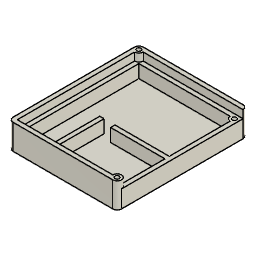
基板外形 (Autodesk Fusion 360 archive; units mm, degrees)
design "筐体A"
Autodesk Fusion 360 part; units mm, degrees
sketch "スケッチ1" plane through (0, 0, 0) normal (0, 0, 1) x (1, 0, 0)
  line L0 (-25, 30) -> (25, 30)
  line L1 (25, 30) -> (25, -30)
  line L2 (25, -30) -> (-25, -30)
  line L3 (-25, -30) -> (-25, 30)
  line L4 (-13.65, 27) -> (13.65, 27)
  line L5 (13.65, 27) -> (13.65, -1.3)
  line L6 (13.65, -1.3) -> (-13.65, -1.3)
  line L7 (-13.65, -1.3) -> (-13.65, 27)
  line L8 (0, 27) -> (0, -1.3)
  line L9 (-7, -6) -> (23, -6)
  line L10 (23, -6) -> (23, -26)
  line L11 (23, -26) -> (-7, -26)
  line L12 (-7, -26) -> (-7, -6)
  line L13 (0, 30) -> (0, -30)
  line L14 (-23, 28) -> (23, 28)
  line L15 (23, 28) -> (23, -28)
  line L16 (23, -28) -> (-23, -28)
  line L17 (-23, -28) -> (-23, 28)
  line L18 (23, 28) -> (25, 28)
  line L19 (23, -28) -> (25, -28)
  circle A0 centre (23, 26) radius 2
  circle A1 centre (23, 26) radius 1
  circle A2 centre (-23, 28) radius 2
  circle A3 centre (-23, 28) radius 1
  circle A4 centre (23, -28) radius 1
  circle A5 centre (23, -28) radius 2
  line L20 (23, -4) -> (-9, -4)
  line L21 (-9, -4) -> (-9, -28)
  line L22 (-9, -28) -> (23, -28)
  line L23 (23, -28) -> (23, -4)
  line L24 (-7, -6) -> (-7, -4)
  line L25 (-2, -6) -> (-2, -4)
  line L26 (-21, 26) -> (23, 26)
  line L27 (23, 26) -> (23, -26)
  line L28 (23, -26) -> (-21, -26)
  line L29 (-21, -26) -> (-21, 26)
  dimension "d1" = 27.3
  dimension "d2" = 28.3
  dimension "d3" = 30
  dimension "d4" = 20
  dimension "d5" = 50
  dimension "d6" = 60
  dimension "d7" = 3
  dimension "d8" = 2
  dimension "d9" = 2
  dimension "d10" = 2
  dimension "d11" = 2
  dimension "d12" = 4
  dimension "d13" = 2
  dimension "d14" = 4
  dimension "d15" = 2
  dimension "d16" = 2
  dimension "d17" = 4
  dimension "d23" = 2
  dimension "d24" = 2
  dimension "d25" = 2
  dimension "d26" = 5
  dimension "d27" = 2
  dimension "d28" = 2
  dimension "d29" = 2
  constraint horizontal L0
  constraint vertical L1
  constraint horizontal L2
  constraint vertical L3
  constraint horizontal L4
  constraint vertical L5
  constraint horizontal L6
  constraint vertical L7
  constraint midpoint L4 L8.start
  constraint midpoint L6 L8.end
  constraint coincident origin L8
  constraint horizontal L9
  constraint vertical L10
  constraint horizontal L11
  constraint vertical L12
  constraint midpoint L0 L13.start
  constraint midpoint L2 L13.end
  constraint midpoint origin L13
  constraint horizontal L14
  constraint vertical L15
  constraint horizontal L16
  constraint vertical L17
  constraint coincident L1 L18.end
  constraint perpendicular L1 L18
  constraint coincident L1 L19.end
  constraint perpendicular L1 L19
  constraint tangent L14 A0
  constraint tangent L1 A0
  constraint concentric A0 A1
  constraint concentric A2 A3
  constraint tangent L0 A2
  constraint tangent L3 A2
  constraint concentric A4 A5
  constraint tangent L1 A5
  constraint tangent L2 A5
  constraint coincident L9.end L15
  constraint horizontal L20
  constraint vertical L21
  constraint horizontal L22
  constraint vertical L23
  constraint coincident L16 L21.end
  constraint coincident L15 L20.start
  constraint coincident L20 L24.end
  constraint perpendicular L20 L24
  constraint coincident L9 L25.start
  constraint coincident L20 L25.end
  constraint perpendicular L20 L25
  constraint horizontal L26
  constraint vertical L27
  constraint horizontal L28
  constraint vertical L29
  constraint collinear L15 L27
  measures "d1" distance of L4.start L4.end
  measures "d2" distance of L4.start L6.end
  measures "d3" distance of L9.start L9.end
  measures "d4" distance of L9.start L11.end
  measures "d5" distance of L0.start L0.end
  measures "d6" distance of L0.end L1.end
  measures "d7" distance of L0 L4
  measures "d8" distance of L3 L17
  measures "d9" distance of L0 L14
  measures "d10" distance of L1 L15
  measures "d11" distance of L2 L16
  measures "d12" diameter of A0
  measures "d13" diameter of A1
  measures "d14" diameter of A2
  measures "d15" diameter of A3
  measures "d16" diameter of A4
  measures "d17" diameter of A5
  measures "d23" distance of L11 L16
  measures "d24" distance of L9 L20
  measures "d25" distance of L12 L21
  measures "d26" distance of L24 L25
  measures "d27" distance of L14 L26
  measures "d28" distance of L17 L29
  measures "d29" distance of L16 L28
extrude "押し出し1" add sketch "スケッチ1" along normal blind 2 contours L0 L13 L14 A2 | L0 L1 L13 L14 L18 | L0 L3 A2 | L14 L17 A2 A3 | L4 L5 L13 L14 A0 L26 | L4 L7 L13 L14 L16 L17 A2 L21 L26 L28 L29 | L1 L18 A0 | L14 L17 A2 A3 | L2 L3 L13 L16 L17 A2 L22 | L4 L7 L8 L13 L26 | L4 L5 L8 L13 L26 | L15 A0 A1 L27 | L15 A0 A1 L26 | L1 L10 L15 A0 A5 L23 L27 | L5 L6 L8 L13 L26 | L6 L7 L8 L13 L26 | L15 A0 A1 L26 L27 | L5 L6 L13 L15 A0 L20 L26 L27 | L16 L19 A4 A5 L22 | L15 L19 A4 A5 L23 | L1 L2 A5 | L2 L13 L16 A5 L22 | L6 L7 L13 L20 L21 L26 L28 L29 | L9 L10 L11 L13 L15 L23 L27 L28 | L11 L13 L16 A5 L22 L28 | L15 L16 A4 A5 L22 L23 | L9 L13 L15 L20 L23 L27 | L11 L13 L16 L21 L22 L28 | L9 L13 L20 L25 | L9 L11 L12 L13 L28 | L12 L20 L21 L24 L28 | L9 L20 L24 L25
extrude "押し出し2" add sketch "スケッチ1" along normal blind 8 contours L0 L13 L14 A2 | L0 L1 L13 L14 L18 | L0 L3 A2 | L14 L17 A2 A3 | L4 L5 L13 L14 A0 L26 | L4 L7 L13 L14 L16 L17 A2 L21 L26 L28 L29 | L1 L18 A0 | L14 L17 A2 A3 | L2 L3 L13 L16 L17 A2 L22 | L4 L7 L8 L13 L26 | L4 L5 L8 L13 L26 | L15 A0 A1 L27 | L15 A0 A1 L26 | L1 L10 L15 A0 A5 L23 L27 | L15 A0 A1 L26 L27 | L16 L19 A4 A5 L22 | L15 L19 A4 A5 L23 | L1 L2 A5 | L2 L13 L16 A5 L22 | L11 L13 L16 A5 L22 L28 | L15 L16 A4 A5 L22 L23 | L9 L13 L15 L20 L23 L27 | L11 L13 L16 L21 L22 L28 | L9 L13 L20 L25 | L12 L20 L21 L24 L28
extrude "押し出し3" add sketch "スケッチ1" along normal blind 11.6 contours L0 L13 L14 A2 | L0 L1 L13 L14 L18 | L0 L3 A2 | L14 L17 A2 A3 | L14 L17 A2 A3 | L2 L3 L13 L16 L17 A2 L22 | L16 L19 A4 A5 L22 | L15 L19 A4 A5 L23 | L1 L2 A5 | L2 L13 L16 A5 L22 | L15 L16 A4 A5 L22 L23
fillet "フィレット1" radius 2 4 edges at (25, -30, 5.8) (-25, -30, 5.8) (25, 30, 5.8) (-25, 30, 5.8)
